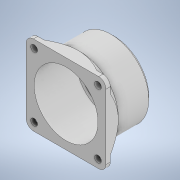
# Autodesk Inventor part: ModuleUSB_Cable
Saved by Autodesk Inventor 2022 (Build 260153000, 153)
## iProperties
Created: 2021-04-23
Part Number: ModuleUSB_Cable
Material: Generic
Document SubType Name: Modeling
Designer: Viktor
Density: 1 g/cm^3
Appearance: Default
Author: Viktor
## iProperties of the stored document ModuleUSB_MINI_3DPrint.ipt
Created: 2021-04-23
Part Number: ModuleUSB_MINI_3DPrint
Material: Generic
Document SubType Name: Modeling
Designer: Viktor
Density: 1 g/cm^3
Appearance: Default
Author: Viktor
Autodesk Inventor part; units mm, degrees
ref_plane "YZ Plane" through (0, 0, 0) normal (1, 0, 0) x (0, 1, 0)
ref_plane "XZ Plane" through (0, 0, 0) normal (0, 1, 0) x (-1, 0, 0)
ref_plane "XY Plane" through (0, 0, 0) normal (0, 0, 1) x (1, 0, 0)
sketch "Sketch1" plane through (0, 0, 0) normal (0, 0, 1) x (1, 0, 0)
  circle A0 centre (0, 0) radius 22
  circle A1 centre (0, 0) radius 26
  dimension "d0" = 44
  dimension "d1" = 4
  constraints: 2 centre point, 2 coincident
  measures "d0" diameter of A0
  measures "d1" radial gap between concentric circles of A0 A1
extrude "Extrusion1" add sketch "Sketch1" along normal blind 30
sketch "Sketch2" plane through (0, 0, 0) normal (0, 0, -1) x (-1, 0, 0)
  circle A0 centre (0, 0) radius 26 projected
extrude "Extrusion2" add sketch "Sketch2" along normal blind 3
sketch "Sketch3" plane through (0, 0, 30) normal (0, 0, 1) x (1, 0, 0)
  circle A0 centre (-22, -22) radius 2.35
  circle A1 centre (0, 0) radius 22 projected
  line L0 (27.5, -27.5) -> (-27.5, -27.5)
  line L1 (-27.5, -27.5) -> (-27.5, 27.5)
  line L2 (-27.5, 27.5) -> (27.5, 27.5)
  line L3 (27.5, 27.5) -> (27.5, -27.5)
  line L4 (27.5, -27.5) -> (-27.5, 27.5) construction
  line L5 (-27.5, -27.5) -> (27.5, 27.5) construction
  circle A2 centre (22, -22) radius 2.35
  circle A3 centre (22, 22) radius 2.35
  circle A4 centre (-22, 22) radius 2.35
  dimension "d6" = 4.7
  dimension "d7" = 22
  dimension "d8" = 22
  dimension "d9" = 55
  dimension "d10" = 55
  dimension "d13" = 360
  constraints: 12 end point, 4 centre point, 2 midpoint, 2 parallel, 1 horizontal, 1 perpendicular, 9 other
  measures "d6" diameter of A0
  measures "d7" horizontal distance of point (0, 0) A0.centre
  measures "d8" horizontal distance of point (0, 0) A0.centre
  measures "d9" distance between parallel lines of L3 L1
  measures "d10" distance between parallel lines of L2 L0
extrude "Extrusion3" add sketch "Sketch3" against normal blind 3
fillet "Fillet1" radius 5 4 edges at (27.5, 27.5, 28.5) (-27.5, 27.5, 28.5) (-27.5, -27.5, 28.5) (27.5, -27.5, 28.5)
chamfer "Chamfer1" distance 7 angle 45 1 edges at (-26, 0, 27)
chamfer "Chamfer2" distance 2 angle 45 1 edges at (26, 0, -3)
sketch "Sketch4" plane through (0, 0, 27) normal (0, 0, -1) x (-1, 0, 0)
  arc A0 (-22.2928, 24.3317) -> (-24.3317, 22.2928) centre (-22, 22) ccw projected
  circle A1 centre (-22, 22) radius 2.35 projected
  line L0 (-18.9381, 25.0619) -> (-17.8174, 20.8793)
  line L1 (-17.8174, 20.8793) -> (-20.8793, 17.8174)
  line L2 (-20.8793, 17.8174) -> (-25.0619, 18.9381)
  line L3 (-25.0619, 18.9381) -> (-26.1826, 23.1207)
  line L4 (-26.1826, 23.1207) -> (-23.1207, 26.1826)
  line L5 (-23.1207, 26.1826) -> (-18.9381, 25.0619)
  line L6 (-27.5, 22.5) -> (-27.5, 18.2414) projected
  circle A2 centre (0, 0) radius 24 projected
  line L7 (-25.0619, -18.9381) -> (-20.8793, -17.8174)
  line L8 (-20.8793, -17.8174) -> (-17.8174, -20.8793)
  line L9 (-17.8174, -20.8793) -> (-18.9381, -25.0619)
  line L10 (-18.9381, -25.0619) -> (-23.1207, -26.1826)
  line L11 (-23.1207, -26.1826) -> (-26.1826, -23.1207)
  line L12 (-26.1826, -23.1207) -> (-25.0619, -18.9381)
  line L13 (18.9381, -25.0619) -> (17.8174, -20.8793)
  line L14 (17.8174, -20.8793) -> (20.8793, -17.8174)
  line L15 (20.8793, -17.8174) -> (25.0619, -18.9381)
  line L16 (25.0619, -18.9381) -> (26.1826, -23.1207)
  line L17 (26.1826, -23.1207) -> (23.1207, -26.1826)
  line L18 (23.1207, -26.1826) -> (18.9381, -25.0619)
  line L19 (25.0619, 18.9381) -> (20.8793, 17.8174)
  line L20 (20.8793, 17.8174) -> (17.8174, 20.8793)
  line L21 (17.8174, 20.8793) -> (18.9381, 25.0619)
  line L22 (18.9381, 25.0619) -> (23.1207, 26.1826)
  line L23 (23.1207, 26.1826) -> (26.1826, 23.1207)
  line L24 (26.1826, 23.1207) -> (25.0619, 18.9381)
  point P0 (-22.2928, -24.3317)
  point P1 (-24.3317, -22.2928)
  point P2 (-22, -22)
  point P3 (-22, -22)
  point P4 (-22, -22)
  point P5 (24.3317, -22.2928)
  point P6 (22.2928, -24.3317)
  point P7 (22, -22)
  point P8 (22, -22)
  point P9 (22, -22)
  point P10 (22.2928, 24.3317)
  point P11 (24.3317, 22.2928)
  point P12 (22, 22)
  point P13 (22, 22)
  point P14 (22, 22)
  dimension "d24" = 135
  dimension "d25" = 7.5
  dimension "d28" = 360
  constraints: 48 end point, 4 coincident, 82 other
  measures "d24" angle of L6 L4
  measures "d25" distance between parallel lines of L1 L4
extrude "Extrusion4" cut sketch "Sketch4" along normal through all contours A1 A0 | L0 L1 L2 L3 L4 L5 | L7 L8 L9 L10 L11 L12 | L13 L14 L15 L16 L17 L18 | L19 L20 L21 L22 L23 L24
sketch "Sketch5" plane through (0, 0, 0) normal (0, 0, 1) x (1, 0, 0)
  circle A0 centre (0, 0) radius 12.5
  dimension "d32" = 25
  constraints: 1 centre point, 1 coincident
  measures "d32" diameter of A0
extrude "Extrusion5" cut sketch "Sketch5" against normal blind 10
chamfer "Chamfer3" distance 1 angle 45 1 edges at (-22, 0, 0)
chamfer "Chamfer4" distance 1 angle 45 1 edges at (-12.5, 0, -3)
equation "\"d8\" = d7"
equation "\"d10\" = d9"
body "Solid1"
